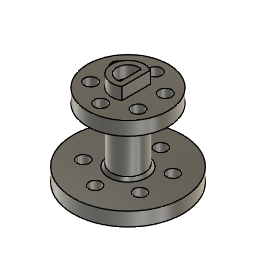
离合拉线盘 v4 (Autodesk Fusion 360 design; units mm, degrees)
Autodesk Fusion 360 part; units mm, degrees
sketch "草图1" plane through (0, 0, 0) normal (0, 0, 1) x (1, 0, 0)
  circle A0 centre (0, 0) radius 20
  circle A1 centre (0, 12) radius 2.25
  circle A2 centre (-10.3923, 6) radius 2.25
  circle A3 centre (-10.3923, -6) radius 2.25
  circle A4 centre (0, -12) radius 2.25
  circle A5 centre (10.3923, -6) radius 2.25
  circle A6 centre (10.3923, 6) radius 2.25
  dimension "d1" = 40
  dimension "d2" = 4.5
  dimension "d3" = 12
  dimension "d5" = 360
  constraint coincident A0.centre origin
  measures "d1" diameter of A0
  measures "d2" diameter of A1
  measures "d3" distance of A0.centre A1.centre
extrude "拉伸1" add sketch "草图1" along normal blind 5
sketch "草图2" plane through (0, 0, 5) normal (0, 0, 1) x (-1, 0, 0)
  circle A0 centre (0, -12) radius 2.25
  circle A1 centre (10.3923, -6) radius 2.25
  circle A2 centre (10.3923, 6) radius 2.25
  circle A3 centre (-10.3923, 6) radius 2.25
  circle A4 centre (0, 12) radius 2.25
  circle A5 centre (-10.3923, -6) radius 2.25
  circle A6 centre (0, 0) radius 20
  circle A7 centre (0, 0) radius 6
  dimension "d8" = 12
  constraint concentric A6 A7
  measures "d8" diameter of A7
extrude "拉伸2" add sketch "草图2" along normal blind 20 contours A7
sketch "草图3" plane through (0, 0, 25) normal (0, 0, 1) x (-1, 0, 0)
  circle A0 centre (0, 0) radius 6
  circle A1 centre (0, 0) radius 40
  circle A2 centre (0, 0) radius 35
  line L0 (11.1263, -33.1844) -> (13, -10)
  line L1 (13, -10) -> (-11.7603, -32.9651)
  line L2 (15.1603, 6.2583) -> (22.6684, -26.6673)
  line L3 (34.3017, -6.9565) -> (15.1603, 6.2583)
  line L4 (2.1603, 16.2583) -> (34.4287, 6.2978)
  line L5 (23.1754, 26.2279) -> (2.1603, 16.2583)
  line L6 (-13, 10) -> (11.7603, 32.9651)
  line L7 (-11.1263, 33.1844) -> (-13, 10)
  line L8 (-15.1603, -6.2583) -> (-22.6684, 26.6673)
  line L9 (-34.3017, 6.9565) -> (-15.1603, -6.2583)
  line L10 (-2.1603, -16.2583) -> (-34.4287, -6.2978)
  line L11 (-23.1754, -26.2279) -> (-2.1603, -16.2583)
  dimension "d11" = 70
  dimension "d12" = 80
  dimension "d14" = 360
  constraint concentric A0 A1
  constraint concentric A1 A2
  constraint coincident A2 L0.start
  constraint coincident A2 L1.end
  measures "d11" diameter of A2
  measures "d12" diameter of A1
sketch "草图4" plane through (0, 0, 25) normal (0, 0, 1) x (-1, 0, 0)
  circle A0 centre (0, 0) radius 14.75
  dimension "d17" = 29.5
  constraint coincident A0.centre origin
  measures "d17" diameter of A0
extrude "拉伸4" add sketch "草图4" along normal blind 5
sketch "草图5" plane through (0, 0, 30) normal (0, 0, 1) x (-1, 0, 0)
  circle A0 centre (0, 0) radius 14.75
  circle A1 centre (0, 0) radius 6
  dimension "d20" = 12
  constraint concentric A0 A1
  measures "d20" diameter of A1
extrude "拉伸5" add sketch "草图5" along normal blind 4.4 contours A1
sketch "草图6" plane through (0, 0, 30) normal (0, 0, 1) x (-1, 0, 0)
  circle A0 centre (0, 0) radius 6
  circle A1 centre (0, 0) radius 14.75
  circle A2 centre (0, -10) radius 2.3
  circle A3 centre (8.6603, -5) radius 2.3
  circle A4 centre (8.6603, 5) radius 2.3
  circle A5 centre (0, 10) radius 2.3
  circle A6 centre (-8.6603, 5) radius 2.3
  circle A7 centre (-8.6603, -5) radius 2.3
  dimension "d23" = 4.6
  dimension "d25" = 360
  dimension "d36" = 10
  dimension "d37" = 10
  measures "d23" diameter of A2
  measures "d36" distance of A0.centre A2.centre
  measures "d37" distance of A0.centre A7.centre
extrude "拉伸6" cut sketch "草图6" against normal blind 10 contours A2 | A3 | A4 | A5 | A6 | A7
sketch "草图7" plane through (0, 0, 34.4) normal (0, 0, 1) x (-1, 0, 0)
  circle A0 centre (0, 0) radius 6
  circle A1 centre (0, 0) radius 6
  circle A2 centre (0, 0) radius 4.5
  line L0 (-3, -6.9008) -> (-3, 8)
  line L1 (-1.5, -6.9008) -> (-1.5, 8)
  dimension "d28" = 1.5
  dimension "d29" = 12
  dimension "d30" = 3
  dimension "d31" = 1.5
  constraint concentric A0 A1
  constraint concentric A1 A2
  constraint vertical L0
  constraint vertical L1
  measures "d28" distance of A1 A2
  measures "d29" diameter of A1
  measures "d30" distance of A0.centre L0
  measures "d31" distance of L0 L1
extrude "拉伸7" cut sketch "草图7" against normal blind 4.4 contours A0 A1 A2 L0 | A2 L1 | A2 L0
chamfer "倒角1" distance 1 angle 45 1 edges at (5.594, -2.1697, 5)
chamfer "倒角2" distance 0.5 angle 45 1 edges at (5.594, 2.1697, 25)
move_face "偏移面1" offset 0.5 2 faces at (-2.5073, -3.7368, 31.4667) (1.5, 1.4142, 32.9333)
